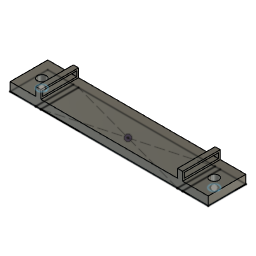
Neopixel Circuit Board (Autodesk Fusion 360 design; units mm, degrees)
Autodesk Fusion 360 part; units mm, degrees
sketch "Sketch1" plane through (0, 0, 0) normal (0, 0, 1) x (1, 0, 0)
  line L0 (40, -11) -> (-40, -11)
  line L1 (-40, -11) -> (-40, 11)
  line L2 (-40, 11) -> (40, 11)
  line L3 (40, 11) -> (40, -11)
  line L4 (40, -11) -> (-40, 11) construction
  line L5 (-40, -11) -> (40, 11) construction
  line L6 (-40, 11) -> (-43, 11)
  line L7 (-43, 11) -> (-43, -11)
  line L8 (-43, -11) -> (-40, -11)
  line L9 (-40, -11) -> (-40, 11)
  line L10 (40, 11) -> (43, 11)
  line L11 (43, 11) -> (43, -11)
  line L12 (43, -11) -> (40, -11)
  line L13 (40, -11) -> (40, 11)
  line L14 (43, 11) -> (58, 11)
  line L15 (58, 11) -> (58, -11)
  line L16 (58, -11) -> (43, -11)
  line L17 (43, -11) -> (43, 11)
  line L18 (-43, 11) -> (-58, 11)
  line L19 (-58, 11) -> (-58, -11)
  line L20 (-58, -11) -> (-43, -11)
  line L21 (-43, -11) -> (-43, 11)
  circle A0 centre (-50.5, 0) radius 2.625
  circle A1 centre (50.5, 0) radius 2.625
  dimension "d1" = 80
  dimension "d2" = 22
  dimension "d3" = 3
  dimension "d4" = 22
  dimension "d5" = 3
  dimension "d6" = 15
  dimension "d7" = 22
  dimension "d8" = 15
  dimension "d9" = 22
  dimension "d10" = 5.25
  dimension "d11" = 5.25
  dimension "d19" = 22
  constraint horizontal L0
  constraint perpendicular L0 L1
  constraint parallel L0 L2
  constraint parallel L1 L3
  constraint coincident L4 origin
  constraint coincident L5 origin
  constraint horizontal L6
  constraint vertical L7
  constraint horizontal L8
  constraint vertical L9
  constraint horizontal L10
  constraint vertical L11
  constraint horizontal L12
  constraint vertical L13
  constraint horizontal L14
  constraint vertical L15
  constraint horizontal L16
  constraint vertical L17
  constraint horizontal L18
  constraint vertical L19
  constraint horizontal L20
  constraint vertical L21
  measures "d1" distance of L1.end L2.end
  measures "d2" distance of L0.end L1.end
  measures "d3" distance of L1.end L6.end
  measures "d4" distance of L1.end L0.end
  measures "d5" distance of L2.end L10.end
  measures "d6" distance of L10.end L14.end
  measures "d7" distance of L10.end L11.end
  measures "d8" distance of L6.end L18.end
  measures "d9" distance of L6.end L7.end
  measures "d10" diameter of A0
  measures "d11" diameter of A1
  measures "d19" distance of L10 L12
extrude "Extrude1" add sketch "Sketch1" along normal blind 5 contours L0 L1 L2 L3 L9 L13 | L11 L14 L15 L16 L17 | L7 L18 L19 L20 L21 makes body 1 at (50.5654, -8.2059, 0) makes body 2 at (13.3333, -3.6667, 0) makes body 3 at (-50.4346, -8.2059, 0)
extrude "Extrude2" add sketch "Sketch1" along normal blind 10 contours L3 L10 L11 L12 L13 L17 | L1 L6 L7 L8 L9 L21 bodies 1 2 3
sketch "Sketch2" plane through (43, 0, 0) normal (1, 0, 0) x (0, 1, 0)
  line L0 (-11, 5) -> (11, 5)
  line L1 (11, 5) -> (11, 10)
  line L2 (11, 10) -> (-11, 10)
  line L3 (-11, 10) -> (-11, 5)
  line L4 (-11, 10) -> (11, 10)
  line L5 (11, 10) -> (11, 5)
  line L6 (11, 5) -> (-11, 5)
  line L7 (-11, 5) -> (-11, 10)
  line L8 (10, 6) -> (-10, 6)
  line L9 (-10, 6) -> (-10, 9)
  line L10 (-10, 9) -> (10, 9)
  line L11 (10, 9) -> (10, 6)
  dimension "d16" = 1
  constraint horizontal L4
  constraint vertical L5
  constraint horizontal L6
  constraint vertical L7
  constraint coincident L0.end L1.start
  constraint coincident L2.end L3.start
  measures "d16" distance of L6
extrude "Extrude3" cut sketch "Sketch2" against normal up to surface (86 mm away) contours L8 L9 L10 L11 bodies 1
equation "d4 = d2"
equation "d7 = d2"
equation "d9 = d2"
equation "d19 = d2"
